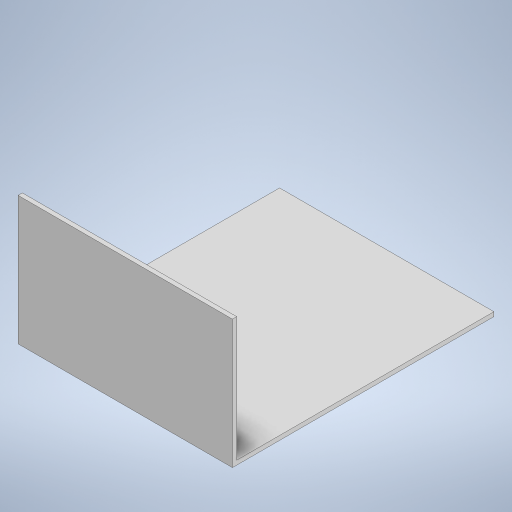
# Autodesk Inventor part: ground
Saved by Autodesk Inventor 2023.2 (Build 272271000, 271)
## iProperties
Created: 2022-11-26
Part Number: ground
Material: Generic
Document SubType Name: Modeling
Designer: omrfrkmll
Density: 1 g/cm^3
Appearance: Default
Author: omrfrkmll
Autodesk Inventor part; units mm, degrees
ref_plane "YZ Plane" through (0, 0, 0) normal (1, 0, 0) x (0, 1, 0)
ref_plane "XZ Plane" through (0, 0, 0) normal (0, 1, 0) x (-1, 0, 0)
ref_plane "XY Plane" through (0, 0, 0) normal (0, 0, 1) x (1, 0, 0)
sketch "Sketch1" plane through (0, 0, 0) normal (0, 1, 0) x (-1, 0, 0)
  line L0 (10.2019, 0) -> (-11.9707, 0)
  line L1 (0, 17.6887) -> (0, -16.1667)
  line L2 (250, 300) -> (-250, 300)
  line L3 (-250, 300) -> (-250, -300)
  line L4 (-250, -300) -> (250, -300)
  line L5 (250, -300) -> (250, 300)
  point P0 (0, 0)
  dimension "d0" = 600
  dimension "d1" = 500
  constraints: 12 end point, 3 horizontal, 2 parallel, 2 vertical, 1 perpendicular, 3 other
  measures "d0" distance between parallel lines of L4 L2
  measures "d1" distance between parallel lines of L3 L5
extrude "Extrusion1" add sketch "Sketch1" along normal blind 10
sketch "Sketch2" plane through (-250, 0, 300) normal (0, 0, 1) x (1, 0, 0)
  line L0 (0, 0) -> (500, 0)
  line L1 (500, 0) -> (500, 300)
  line L2 (500, 300) -> (0, 300)
  line L3 (0, 300) -> (0, 0)
  point P0 (250, 0)
  dimension "d4" = 300
  dimension "d5" = 500
  constraints: 8 end point, 2 parallel, 1 horizontal, 1 perpendicular
  measures "d4" distance between parallel lines of L0 L2
  measures "d5" distance between parallel lines of L3 L1
extrude "Extrusion2" add sketch "Sketch2" along normal blind 10
body "Solid1"
